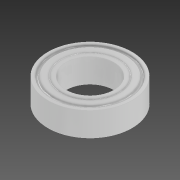
# Autodesk Inventor part: lager 8mm - buiten 14 (sven 2 stuks)
Saved by Autodesk Inventor 2020 (Build 240168000, 168)
## iProperties
Created: 2020-05-19
Part Number: lager 8mm - buiten 14 (sven 2 stuks)
Material: Generic
Document SubType Name: Modeling
Designer: stefa
Density: 1 g/cm^3
Appearance: Aluminum - Polished
Author: stefa
Autodesk Inventor part; units mm, degrees
ref_plane "YZ Plane" through (0, 0, 0) normal (1, 0, 0) x (0, 1, 0)
ref_plane "XZ Plane" through (0, 0, 0) normal (0, 1, 0) x (-1, 0, 0)
ref_plane "XY Plane" through (0, 0, 0) normal (0, 0, 1) x (1, 0, 0)
sketch "Sketch1" plane through (0, 0, 0) normal (0, 0, 1) x (1, 0, 0)
  line L0 (-7, 2) -> (-4, 2)
  line L1 (-4, 2) -> (-4, 0)
  line L2 (-4, 0) -> (-7, 0)
  line L3 (-7, 0) -> (-7, 2)
  circle A0 centre (-6.2, 2) radius 0.25
  circle A1 centre (-4.8, 2) radius 0.1
  line L4 (0, -3.15) -> (0, 3.15) projected
  line L5 (0, 0) -> (-13.6297, 0) construction
  line L6 (-7, -2) -> (-4, -2)
  line L7 (-4, -2) -> (-4, 0)
  line L8 (-7, 0) -> (-7, -2)
  circle A2 centre (-6.2, -2) radius 0.25
  circle A3 centre (-4.8, -2) radius 0.1
  point P0 (-4.7, 2)
  point P1 (-4.9, 2)
  point P2 (-5.95, 2)
  point P3 (-6.45, 2)
  point P4 (-6.45, -2)
  point P5 (-5.95, -2)
  point P6 (-4.9, -2)
  point P7 (-4.7, -2)
  dimension "d0" = 2
  dimension "d1" = 4
  dimension "d2" = 7
  dimension "d3" = 0.5
  dimension "d4" = 0.2
  dimension "d5" = 0.8
  dimension "d6" = 2.2
  constraints: 16 end point, 5 point on line, 4 centre point, 4 symmetric about line, 2 horizontal, 2 parallel, 1 perpendicular, 2 other
  measures "d0" distance of L2.end L0.start
  measures "d1" distance from line of L5.start L1
  measures "d2" distance from line of L5.start L3
  measures "d3" diameter of A0
  measures "d4" diameter of A1
  measures "d5" distance from line of L1 A1.centre
  measures "d6" distance from line of L1 A0.centre
revolve "Revolution1" add sketch "Sketch1" angle 360 about axis through (0, -10, 0) along (0, 1, 0) contours L0 L1 L2 L3 A0 A1 | L7 L6 A3 A2 L8 L2
body "Solid1"
